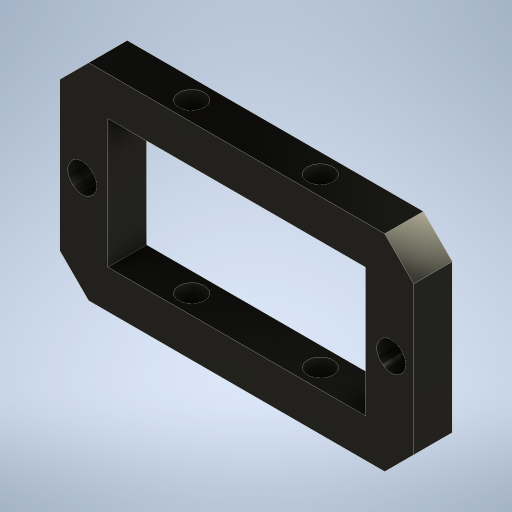
# Autodesk Inventor part: ServoCarrier
Saved by Autodesk Inventor 2024.3 (Build 283343000, 343)
## iProperties
Created: 2025-01-07
Part Number: ServoCarrier
Material: Generic
Document SubType Name: Modeling
Designer: migue
Density: 1 g/cm^3
Appearance: Gunmetal
Author: migue
Autodesk Inventor part; units mm, degrees
ref_plane "YZ Plane" through (0, 0, 0) normal (1, 0, 0) x (0, 1, 0)
ref_plane "XZ Plane" through (0, 0, 0) normal (0, 1, 0) x (-1, 0, 0)
ref_plane "XY Plane" through (0, 0, 0) normal (0, 0, 1) x (1, 0, 0)
sketch "Sketch1" plane through (0, 0, 0) normal (0, 0, 1) x (1, 0, 0)
  line L0 (-20, 10) -> (20, 10)
  line L1 (20, 10) -> (20, -10)
  line L2 (20, -10) -> (-20, -10)
  line L3 (-20, -10) -> (-20, 10)
  line L4 (-20, 10) -> (20, -10) construction
  line L5 (20, 10) -> (-20, -10) construction
  line L6 (-27.5, 16) -> (27.5, 16)
  line L7 (27.5, 16) -> (27.5, -16)
  line L8 (27.5, -16) -> (-27.5, -16)
  line L9 (-27.5, -16) -> (-27.5, 16)
  line L10 (-27.5, 16) -> (27.5, -16) construction
  line L11 (27.5, 16) -> (-27.5, -16) construction
  line L12 (0, 0) -> (0, 16) construction
  circle A0 centre (-24, 0) radius 2.25
  circle A1 centre (24, 0) radius 2.25
  dimension "d0" = 40
  dimension "d1" = 20
  dimension "d2" = 32
  dimension "d3" = 55
  dimension "d4" = 4.5
  dimension "d5" = 24
  constraints: 26 end point, 5 midpoint, 4 parallel, 2 centre point, 2 horizontal, 2 perpendicular, 1 symmetric about line, 1 other
  measures "d0" distance of L0.start L0.end
  measures "d1" distance of L0.end L1.end
  measures "d2" distance of L6.end L7.end
  measures "d3" distance of L6.start L6.end
  measures "d4" diameter of A0
  measures "d5" distance of A0.centre L12.start
extrude "Extrusion1" add sketch "Sketch1" along normal blind 6
chamfer "Chamfer1" distance 4.5 angle 45 4 edges at (27.5, 16, 3) (27.5, -16, 3) (-27.5, -16, 3) (-27.5, 16, 3)
sketch "Sketch2" plane through (-23, 16, 0) normal (0, 1, 0) x (1, 0, 0)
  line L0 (50.5, -6) -> (50.5, 0) projected
  line L1 (50.5, -3) -> (-4.5, -3) construction
  line L2 (-4.5, 0) -> (-4.5, -6) projected
  line L3 (23, 0) -> (23, -6) construction
  circle A0 centre (33, -3) radius 2
  circle A1 centre (13, -3) radius 2
  dimension "d11" = 10
  dimension "d12" = 4
  constraints: 4 end point, 2 centre point, 2 midpoint, 1 point on line, 1 symmetric about line, 1 vertical, 1 other
  measures "d11" distance from line of A0.centre L3
  measures "d12" diameter of A0
extrude "Extrusion2" cut sketch "Sketch2" against normal through all
body "Solid1"
